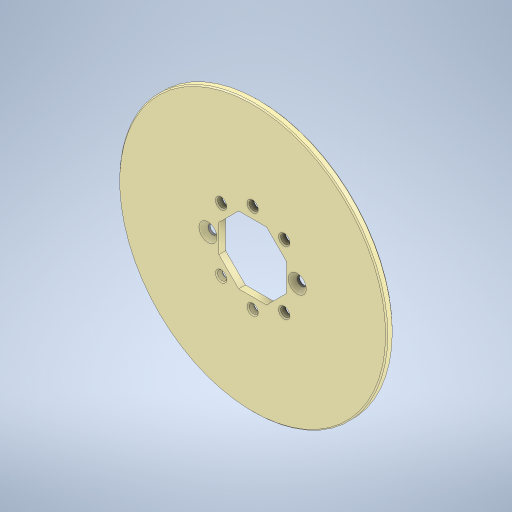
# Autodesk Inventor part: spool_side
Saved by Autodesk Inventor 2023.4 (Build 274418000, 418)
## iProperties
Created: 2023-11-23
Part Number: spool_side
Material: Generic
Document SubType Name: Modeling
Designer: aaron
Density: 1 g/cm^3
Appearance: Default
Author: aaron
Autodesk Inventor part; units mm, degrees
ref_plane "YZ Plane" through (0, 0, 0) normal (1, 0, 0) x (0, 1, 0)
ref_plane "XZ Plane" through (0, 0, 0) normal (0, 1, 0) x (-1, 0, 0)
ref_plane "XY Plane" through (0, 0, 0) normal (0, 0, 1) x (1, 0, 0)
sketch "Sketch1" plane through (0, 0, 0) normal (0, 0, 1) x (1, 0, 0)
  circle A0 centre (0, 0) radius 60
  dimension "d0" = 120
  constraints: 1 centre point, 1 coincident
  measures "d0" diameter of A0
extrude "Extrusion1" add sketch "Sketch1" along normal blind 3
sketch "Sketch3" plane through (0, 0, 3) normal (0, 0, 1) x (1, 0, 0)
  line L0 (-15.1, 6.2546) -> (-6.2546, 15.1)
  line L1 (-15.1, -6.2546) -> (-15.1, 6.2546)
  line L2 (-6.2546, -15.1) -> (-15.1, -6.2546)
  line L3 (6.2546, -15.1) -> (-6.2546, -15.1)
  line L4 (15.1, -6.2546) -> (6.2546, -15.1)
  line L5 (15.1, 6.2546) -> (15.1, -6.2546)
  line L6 (6.2546, 15.1) -> (15.1, 6.2546)
  line L7 (-6.2546, 15.1) -> (6.2546, 15.1)
  point P0 (0, 0)
  point P1 (0, 0)
  constraints: 16 end point
extrude "Extrusion3" cut sketch "Sketch3" against normal through all
sketch "Sketch4" plane through (0, 0, 3) normal (0, 0, 1) x (1, 0, 0)
  line L0 (0, 0) -> (41.4197, 0)
  circle A0 centre (20, 0) radius 2.05
  circle A1 centre (20, 0) radius 2.05
  circle A2 centre (14.1421, 14.1421) radius 2.05
  circle A3 centre (0, 20) radius 2.05
  circle A4 centre (-14.1421, 14.1421) radius 2.05
  circle A5 centre (-20, 0) radius 2.05
  circle A6 centre (-14.1421, -14.1421) radius 2.05
  circle A7 centre (0, -20) radius 2.05
  circle A8 centre (14.1421, -14.1421) radius 2.05
  dimension "d26" = 360
  dimension "d27" = 4.1
  constraints: 9 centre point, 2 end point, 1 coincident, 1 concentric, 1 horizontal, 17 other
  measures "d27" diameter of A0
extrude "Extrusion4" cut sketch "Sketch4" against normal through all
chamfer "Chamfer1" distance 2 angle 45 2 edges at (-22.05, 0, 3) (17.95, 0, 3)
chamfer "Chamfer2" distance 0.5 angle 45 14 edges at (-60, 0, 3) (-60, 0, 0) (-2.05, -20, 3) (12.0921, -14.1421, 3) (-16.1921, -14.1421, 3) (-16.1921, 14.1421, 3) (-2.05, 20, 3) (12.0921, 14.1421, 3) (-16.1921, -14.1421, 0) (-2.05, -20, 0) (12.0921, -14.1421, 0) (-16.1921, 14.1421, 0) (-2.05, 20, 0) (12.0921, 14.1421, 0)
body "Solid1"
